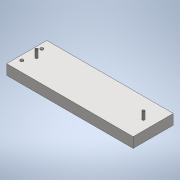
# Autodesk Inventor part: resistencia_cuarzo_550W
Saved by Autodesk Inventor 2021 (Build 250183000, 183)
## iProperties
Created: 2021-04-16
Part Number: resistencia_cuarzo_550W
Material: Genérico
Document SubType Name: Modeling
Designer: Leonardo Fabio Mercado Benítez
Density: 1 g/cm^3
Appearance: Valor por defecto
Categories: <MemberInstance><Categories><Category DisplayName="" Mnemonic="CABLEANDHARNESS" InternalName="e4a7e005-5e42-4d16-b293-125e7f0d0512"><Category DisplayName="" Mnemonic="CONNECTORS" InternalName="6f634eba-a678-4820-a31d-2c2d5ee6728e"><CategoryParameter DisplayName="" Mnemonic="REFDES" InternalName="c3740e8c-60ab-4d5d-8584-52b73222f2f0"/><Category DisplayName="" Mnemonic="DISCRETEWIRE" InternalName="9a3407de-09b2-4cdb-8c40-9708d5144a28"/></Category></Category></Categories><FamilyTemplate><FamilyTemplateParameters></FamilyTemplateParameters></FamilyTemplate><CategoryParameterMap><ParamToTemplateMap><ParamToTemplate CategoryParameter="//CategoryParameter[@InternalName='c3740e8c-60ab-4d5d-8584-52b73222f2f0']" ConstantValue=""/></ParamToTemplateMap></CategoryParameterMap></MemberInstance>
Author: Leonardo Fabio Mercado Benítez
Autodesk Inventor part; units mm, degrees
ref_plane "YZ Plane" through (0, 0, 0) normal (1, 0, 0) x (0, 1, 0)
ref_plane "XZ Plane" through (0, 0, 0) normal (0, 1, 0) x (-1, 0, 0)
ref_plane "XY Plane" through (0, 0, 0) normal (0, 0, 1) x (1, 0, 0)
sketch "Boceto1" plane through (0, 0, 0) normal (0, 1, 0) x (-1, 0, 0)
  line L0 (-157.5, 50) -> (157.5, 50)
  line L1 (157.5, 50) -> (157.5, -50)
  line L2 (157.5, -50) -> (-157.5, -50)
  line L3 (-157.5, -50) -> (-157.5, 50)
  line L4 (-157.5, 50) -> (157.5, -50) construction
  line L5 (157.5, 50) -> (-157.5, -50) construction
  point P0 (0, 0)
  dimension "d0" = 315
  dimension "d1" = 100
  constraints: 12 end point, 2 midpoint, 2 parallel, 1 horizontal, 1 perpendicular
  measures "d0" distance of L1.end L2.end
  measures "d1" distance of L0.end L1.end
extrude "Extrusión1" add sketch "Boceto1" along normal blind 25.4
sketch "Boceto2" plane through (0, 0, 0) normal (0, -1, 0) x (1, 0, 0)
  line L0 (-144.8, 48.98) -> (144.8, 48.98)
  line L1 (144.8, -48.98) -> (-144.8, -48.98)
  line L2 (-144.8, -48.98) -> (-144.8, 48.98)
  line L3 (144.8, 48.98) -> (144.8, -48.98)
  line L4 (-157.5, -50) -> (-157.5, 50) projected
  line L5 (-157.5, 50) -> (157.5, 50) projected
  line L6 (157.5, 50) -> (157.5, -50) projected
  dimension "d8" = 12.7
  dimension "d9" = 1.02
  dimension "d52" = 12.7
  constraints: 8 end point
  measures "d8" distance between parallel lines of L4 L2
  measures "d9" distance between parallel lines of L5 L0
  measures "d52" distance between parallel lines of L3 L6
extrude "Extrusión2" cut sketch "Boceto2" against normal blind 24.38
sketch "Boceto4" plane through (0, 25.4, 0) normal (0, 1, 0) x (1, 0, 0)
  line L0 (-157.5, 50) -> (-108.5, 50) construction
  line L1 (-108.5, 50) -> (-108.5, -50) construction
  line L2 (-157.5, -50) -> (157.5, -50) construction
  line L3 (-157.5, -50) -> (-108.5, 50) construction
  line L4 (-157.5, 50) -> (-108.5, -50) construction
  line L5 (157.5, 50) -> (-157.5, 50) construction
  line L6 (157.5, 50) -> (108.5, 50) construction
  line L7 (108.5, 50) -> (108.5, -50) construction
  line L8 (108.5, -50) -> (157.5, 50) construction
  line L9 (108.5, 50) -> (157.5, -50) construction
  circle A0 centre (-133, 0) radius 3.175
  circle A1 centre (133, 0) radius 3.175
  point P0 (0, 0)
  dimension "d24" = 49
  dimension "d25" = 49
  dimension "d26" = 6.35
  dimension "d27" = 6.35
  constraints: 16 end point, 3 perpendicular, 3 point on line, 2 centre point, 2 midpoint
  measures "d24" distance of L0.start L0.end
  measures "d25" distance of L5.start L6.end
  measures "d26" diameter of A0
  measures "d27" diameter of A1
extrude "Extrusión4" add sketch "Boceto4" along normal blind 19.05
thread "Rosca1" size "1/4-20 UNC" class "1A" standard "ANSI Unified Screw Threads" full length
thread "Rosca2" size "M7x1" class "6g" standard "ANSI Metric M Profile" full length
chamfer "Chaflán1" distance 0.5 angle 45 1 edges at (-136.175, 44.45, 0)
chamfer "Chaflán2" distance 0.5 angle 45 1 edges at (129.825, 44.45, 0)
sketch "Boceto6" plane through (-144.8, 0, 48.98) normal (1, 0, 0) x (0, 0, -1)
  circle A0 centre (7, 6.35) radius 4.7625
  line L0 (0, 0) -> (0, 24.38) projected
  line L1 (97.96, 0) -> (0, 0) projected
  circle A1 centre (17.5, 6.35) radius 4.7625
  circle A2 centre (28, 6.35) radius 4.7625
  circle A3 centre (38.5, 6.35) radius 4.7625
  circle A4 centre (49, 6.35) radius 4.7625
  circle A5 centre (59.5, 6.35) radius 4.7625
  circle A6 centre (70, 6.35) radius 4.7625
  circle A7 centre (80.5, 6.35) radius 4.7625
  circle A8 centre (91, 6.35) radius 4.7625
  point P0 (48.98, 0)
  dimension "d53" = 9.525
  dimension "d54" = 7
  dimension "d55" = 6.35
  dimension "d58" = 10.5
  constraints: 9 centre point, 1 horizontal, 16 other
  measures "d53" diameter of A0
  measures "d54" distance from line of L0 A0.centre
  measures "d55" distance from line of L1 A0.centre
  measures "d58" distance of A0.centre A1.centre
extrude "Extrusión6" add sketch "Boceto6" along normal up to surface (289.6 mm away)
sketch "Boceto7" plane through (0, 25.4, 0) normal (0, 1, 0) x (1, 0, 0)
  line L0 (-157.5, 50) -> (-157.5, -50) construction
  line L1 (-157.5, 0) -> (-144.8, 0) construction
  line L2 (-144.8, 0) -> (-144.8, 25) construction
  line L3 (-144.8, 48.98) -> (-144.8, -48.98) construction
  line L4 (-144.8, 0) -> (-144.8, -25) construction
  circle A0 centre (-144.8, -25) radius 3.175
  circle A1 centre (-144.8, 25) radius 3.175
  circle A2 centre (-144.8, -25) radius 3.685
  circle A3 centre (-144.8, 25) radius 3.685
  point P0 (0, 0)
  dimension "d67" = 12.7
  dimension "d68" = 25
  dimension "d69" = 25
  dimension "d70" = 6.35
  dimension "d71" = 6.35
  dimension "d72" = 7.37
  dimension "d73" = 7.37
  constraints: 6 end point, 4 centre point, 4 coincident, 2 point on line, 1 horizontal, 1 midpoint
  measures "d67" distance of L1.start L1.end
  measures "d68" distance of L1.end L2.end
  measures "d69" distance of L1.end L4.end
  measures "d70" diameter of A0
  measures "d71" diameter of A1
  measures "d72" diameter of A2
  measures "d73" diameter of A3
extrude "Extrusión7" add sketch "Boceto7" along normal blind 2
chamfer "Chaflán4" distance 0.5 angle 45 2 edges at (-148.485, 27.4, 25) (-148.485, 27.4, -25)
sketch "Boceto8" plane through (-144.8, 25.4, -25) normal (0, 1, 0) x (1, 0, 0)
  circle A0 centre (0, 0) radius 3.175 projected
sketch "Boceto9" plane through (-144.8, 25.4, 25) normal (0, 1, 0) x (1, 0, 0)
  circle A0 centre (0, 0) radius 3.175 projected
